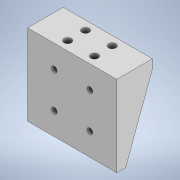
# Autodesk Inventor part: 線性滑塊轉接器
Saved by Autodesk Inventor 2021 (Build 250183000, 183)
## iProperties
Created: 2023-02-14
Part Number: 線性滑塊轉接器
Material: 一般
Document SubType Name: Modeling
Designer: brian
Density: 1 g/cm^3
Appearance: 預設
Author: brian
Autodesk Inventor part; units mm, degrees
ref_plane "YZ Plane" through (0, 0, 0) normal (1, 0, 0) x (0, 1, 0)
ref_plane "XZ Plane" through (0, 0, 0) normal (0, 1, 0) x (-1, 0, 0)
ref_plane "XY Plane" through (0, 0, 0) normal (0, 0, 1) x (1, 0, 0)
sketch "草圖1" plane through (0, 0, 0) normal (1, 0, 0) x (0, 1, 0)
  line L0 (0, 0) -> (45.4, 0)
  line L1 (45.4, 0) -> (45.4, -20)
  line L2 (45.4, -20) -> (40.4, -20)
  line L3 (40.4, -20) -> (0, -5)
  line L4 (0, -5) -> (0, 0)
  dimension "d0" = 45.4
  dimension "d1" = 20
  dimension "d2" = 5
  dimension "d3" = 5
  constraints: 10 end point, 2 perpendicular, 1 horizontal, 1 parallel
  measures "d0" distance of L0.start L0.end
  measures "d1" distance of L0.end L1.end
  measures "d2" distance of L1.end L2.end
  measures "d3" distance of L3.end L0.start
extrude "擠出1" add sketch "草圖1" along normal mid plane 50
sketch "草圖2" plane through (25, 45.4, -20) normal (0, 0, -1) x (-1, 0, 0)
  line L0 (15, -12.7) -> (35, -12.7)
  line L1 (35, -12.7) -> (35, -32.7)
  line L2 (35, -32.7) -> (15, -32.7)
  line L3 (15, -32.7) -> (15, -12.7)
  line L4 (15, -12.7) -> (35, -32.7) construction
  line L5 (35, -12.7) -> (15, -32.7) construction
  line L6 (0, 0) -> (0, -45.4) projected
  point P0 (25, -45.4)
  point P1 (25, -22.7)
  point P2 (25, -22.7)
  point P3 (25, -22.7)
  point P4 (0, -22.7)
  dimension "d6" = 20
  dimension "d7" = 20
  constraints: 12 end point, 5 midpoint, 4 coincident, 2 parallel, 1 horizontal, 1 horizontal alignment, 1 perpendicular, 1 vertical alignment
  measures "d6" distance of L1.end L2.end
  measures "d7" distance of L0.end L1.end
hole "孔1" at (10, 32.7, -20) at (10, 12.7, -20) at (-10, 12.7, -20) at (-10, 32.7, -20) direction (0, 0, 1) diameter 3.2 end through all counterbore diameter 5.7 counterbore depth 15
sketch "草圖3" plane through (-25, 45.4, 0) normal (0, 1, 0) x (1, 0, 0)
  line L0 (32.5, 15) -> (17.5, 15)
  line L1 (17.5, 15) -> (17.5, 5)
  line L2 (17.5, 5) -> (32.5, 5)
  line L3 (32.5, 5) -> (32.5, 15)
  line L4 (32.5, 15) -> (17.5, 5) construction
  line L5 (17.5, 15) -> (32.5, 5) construction
  line L6 (0, 0) -> (0, 20) projected
  line L7 (0, 20) -> (50, 20) projected
  point P0 (25, 0)
  point P1 (25, 10)
  point P2 (25, 10)
  point P3 (0, 10)
  point P4 (25, 10)
  point P5 (25, 20)
  dimension "d15" = 15
  dimension "d16" = 10
  constraints: 12 end point, 6 midpoint, 4 coincident, 2 parallel, 1 horizontal, 1 horizontal alignment, 1 perpendicular, 1 vertical alignment
  measures "d15" distance of L2.end L1.end
  measures "d16" distance of L1.end L0.end
hole "孔2" at (7.5, 45.4, -5) at (-7.5, 45.4, -5) at (-7.5, 45.4, -15) at (7.5, 45.4, -15) direction (0, -1, 0) diameter 2.7 depth 10 counterbore diameter 4.1 counterbore depth 6
equation "\"d3\" = d2"
